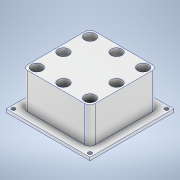
# Autodesk Inventor part: Aluminium Container 0805
Saved by Autodesk Inventor 2020 (Build 240168000, 168)
## iProperties
Created: 2022-07-27
Part Number: Aluminium Container 0805
Material: Aluminum 6061
Document SubType Name: Modeling
Designer: Administrator
Density: 2.7 g/cm^3
Appearance: Aluminum - Flat
Author: Administrator
Autodesk Inventor part; units mm, degrees
ref_plane "YZ Plane" through (0, 0, 0) normal (1, 0, 0) x (0, 1, 0)
ref_plane "XZ Plane" through (0, 0, 0) normal (0, 1, 0) x (-1, 0, 0)
ref_plane "XY Plane" through (0, 0, 0) normal (0, 0, 1) x (1, 0, 0)
sketch "Sketch1" plane through (0, 0, 0) normal (0, 1, 0) x (-1, 0, 0)
  line L0 (28, 33) -> (-28, 33)
  line L1 (-33, 28) -> (-33, -28)
  line L2 (-28, -33) -> (28, -33)
  line L3 (33, -28) -> (33, 28)
  line L4 (33, 33) -> (-33, -33) construction
  line L5 (-33, 33) -> (33, -33) construction
  arc A0 (28, -33) -> (33, -28) centre (28, -28) ccw
  arc A1 (33, 28) -> (28, 33) centre (28, 28) ccw
  arc A2 (-28, 33) -> (-33, 28) centre (-28, 28) ccw
  arc A3 (-33, -28) -> (-28, -33) centre (-28, -28) ccw
  point P0 (0, 0)
  dimension "d0" = 66
  dimension "d1" = 66
  dimension "d4" = 5
  constraints: 12 end point, 8 point on circle, 8 point on line, 8 tangent, 4 centre point, 3 equal radius, 2 midpoint, 2 parallel, 1 horizontal, 1 perpendicular
  measures "d0" distance of L5.end L4.end
  measures "d1" distance of L4.end L5.start
  measures "d4" radius of A0
extrude "Extrusion1" add sketch "Sketch1" along normal blind 35
sketch "Sketch2" plane through (0, 35, 0) normal (0, 1, 0) x (1, 0, 0)
  line L0 (0, 0) -> (-10, 0)
  line L1 (0, 0) -> (0, -10)
  circle A0 centre (26, 26) radius 5.35
  circle A1 centre (0, 26) radius 5.35
  circle A2 centre (-26, 26) radius 5.35
  circle A3 centre (26, 0) radius 5.35
  circle A4 centre (0, 0) radius 5.35
  circle A5 centre (-26, 0) radius 5.35
  circle A6 centre (26, -26) radius 5.35
  circle A7 centre (0, -26) radius 5.35
  circle A8 centre (-26, -26) radius 5.35
  dimension "d8" = 10
  dimension "d9" = 10
  dimension "d10" = 10.7
  dimension "d11" = 26
  dimension "d12" = 26
  dimension "d15" = 26
  dimension "d18" = 26
  constraints: 9 centre point, 4 end point, 2 horizontal, 2 vertical, 16 other
  measures "d8" distance of L0.start L0.end
  measures "d9" distance of L0.start L1.end
  measures "d10" diameter of A0
  measures "d11" distance from line of L1 A0.centre
  measures "d12" distance from line of L0 A0.centre
  measures "d15" distance of A0.centre A1.centre
  measures "d18" distance of A0.centre A3.centre
extrude "Extrusion2" cut sketch "Sketch2" against normal blind 35 contours A0 | A1 | A2 | A3 | A5 | A6 | A7 | A8
sketch "Sketch4" plane through (0, 0, 0) normal (0, -1, 0) x (1, 0, 0)
  line L0 (37.5, 37.5) -> (-37.5, -37.5) construction
  line L1 (-37.5, 37.5) -> (37.5, -37.5) construction
  line L2 (-41, -38) -> (-41, 38)
  line L3 (41, -41) -> (-41, 41) construction
  line L4 (-41, -41) -> (41, 41) construction
  circle A0 centre (-37.5, 37.5) radius 1.85
  line L5 (38, 41) -> (-38, 41)
  line L6 (-38, -41) -> (38, -41)
  line L7 (41, -38) -> (41, 38)
  line L8 (41, 41) -> (-41, -41) construction
  line L9 (-41, 41) -> (41, -41) construction
  circle A1 centre (-37.5, -37.5) radius 1.85
  circle A2 centre (37.5, 37.5) radius 1.85
  circle A3 centre (37.5, -37.5) radius 1.85
  line L10 (-41, -38) -> (-41, -41)
  line L11 (-38, -41) -> (-41, -41)
  line L12 (-41, 38) -> (-41, 41)
  line L13 (-38, 41) -> (-41, 41)
  line L14 (38, 41) -> (41, 41)
  line L15 (41, 38) -> (41, 41)
  line L16 (41, -38) -> (41, -41)
  line L17 (41, -41) -> (38, -41)
  point P0 (0, 0)
  dimension "d28" = 75
  dimension "d29" = 75
  dimension "d31" = 82
  dimension "d56" = 3.7
  dimension "d68" = 75
  dimension "d71" = 75
  constraints: 36 end point, 6 midpoint, 6 point on line, 4 centre point, 3 collinear, 3 perpendicular, 3 vertical, 2 horizontal, 1 coincident, 1 parallel, 6 other
  measures "d28" distance of L1.end L0.end
  measures "d29" distance of L0.end L1.start
  measures "d31" distance of L4.start L3.end
  measures "d56" diameter of A0
  measures "d68" distance of A0.centre A1.centre
  measures "d71" distance of A0.centre A2.centre
extrude "Extrusion4" add sketch "Sketch4" along normal blind 3
thread "Thread5" size "M3.5x0.6" class "6H" standard "ANSI Metric M Profile" length 5.5
thread "Thread6" size "M3.5x0.6" class "6H" standard "ANSI Metric M Profile" length 5.5
thread "Thread7" size "M3.5x0.6" class "6H" standard "ANSI Metric M Profile" length 5.5
thread "Thread8" size "M3.5x0.6" class "6H" standard "ANSI Metric M Profile" length 5.5
body "Solid1"
